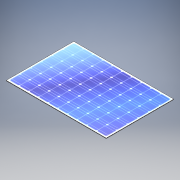
# Autodesk Inventor part: Solar Panel
Saved by Autodesk Inventor 2017 (Build 210142000, 142)
## iProperties
Created: 2021-04-11
Part Number: Solar Panel
Material: ABS Plastic
Document SubType Name: Modeling
Designer: udays
Density: 1.06 g/cm^3
Appearance: Smooth - White
Author: udays
Autodesk Inventor part; units mm, degrees
ref_plane "YZ Plane" through (0, 0, 0) normal (1, 0, 0) x (0, 1, 0)
ref_plane "XZ Plane" through (0, 0, 0) normal (0, 1, 0) x (-1, 0, 0)
ref_plane "XY Plane" through (0, 0, 0) normal (0, 0, 1) x (1, 0, 0)
sketch "Sketch1" plane through (0, 0, 0) normal (0, 1, 0) x (-1, 0, 0)
  line L0 (0, 0) -> (635.6191, -1.147) construction
  line L1 (635.6191, -1.147) -> (634.8468, -429.1305) construction
  line L2 (634.8468, -429.1305) -> (-0.7723, -427.9835) construction
  line L3 (-0.7723, -427.9835) -> (0, 0) construction
  constraints: 2 other
sketch "Sketch2" plane through (0, 0, 0) normal (0, 1, 0) x (-1, 0, 0)
  line L0 (0, 0) -> (634.9168, 0)
  line L1 (634.9168, 0) -> (634.9168, -429.2244)
  line L2 (634.9168, -429.2244) -> (0, -429.2244)
  line L3 (0, -429.2244) -> (0, 0)
  dimension "d8" = 429.2244
  dimension "d9" = 634.9168
  constraints: 8 end point, 2 parallel, 1 horizontal, 1 perpendicular
  measures "d8" distance of L0.end L1.end
  measures "d9" distance of L1.end L2.end
extrude "Extrusion1" add sketch "Sketch2" against normal blind 3.175
decal "Decal1"
chamfer "Chamfer1" distance 0.635 angle 45 8 edges at (-317.4584, 0, 0) (0, 0, -214.6122) (-317.4584, 0, -429.2244) (-634.9168, 0, -214.6122) (0, -1.5875, 0) (0, -1.5875, -429.2244) (-634.9168, -1.5875, 0) (-634.9168, -1.5875, -429.2244)
fillet "Fillet1" radius 0.635 8 edges at (-317.4584, -3.175, -429.2244) (-0.3175, -3.175, -428.9069) (0, -3.175, -214.6122) (-0.3175, -3.175, -0.3175) (-317.4584, -3.175, 0) (-634.5993, -3.175, -0.3175) (-634.9168, -3.175, -214.6122) (-634.5993, -3.175, -428.9069)
fillet "Fillet2" radius 0.0254 36 edges at (-0.635, -1.5875, 0) (-317.4584, -0.635, 0) (-634.2818, -1.5875, 0) (0, -1.5875, -0.635) (-0.3175, -0.635, -0.3175) (-0.712, -2.989, -0.186) (-634.2048, -2.989, -0.186) (-0.635, -0.3175, -0.3175) (-634.2818, -0.3175, -0.3175) (-317.4584, 0, -0.635) (-634.9168, -1.5875, -0.635) (-634.5993, -0.635, -0.3175) (0, -1.5875, -428.5894) (0, -0.635, -214.6122) (-0.186, -2.989, -0.712) (-0.3175, -0.3175, -0.635) (-634.7309, -2.989, -0.712) (-634.5993, -0.3175, -0.635) (-0.635, 0, -214.6122) (-634.2818, 0, -214.6122) (-317.4584, 0, -428.5894) (-634.9168, -0.635, -214.6122) (-634.9168, -1.5875, -428.5894) (-0.635, -1.5875, -429.2244) (-0.3175, -0.635, -428.9069) (-0.186, -2.989, -428.5124) (-0.3175, -0.3175, -428.5894) (-634.2048, -2.989, -429.0385) (-0.712, -2.989, -429.0385) (-634.7309, -2.989, -428.5124) (-634.5993, -0.3175, -428.5894) (-317.4584, -0.635, -429.2244) (-634.2818, -0.3175, -428.9069) (-0.635, -0.3175, -428.9069) (-634.5993, -0.635, -428.9069) (-634.2818, -1.5875, -429.2244)
body "Solid1"
